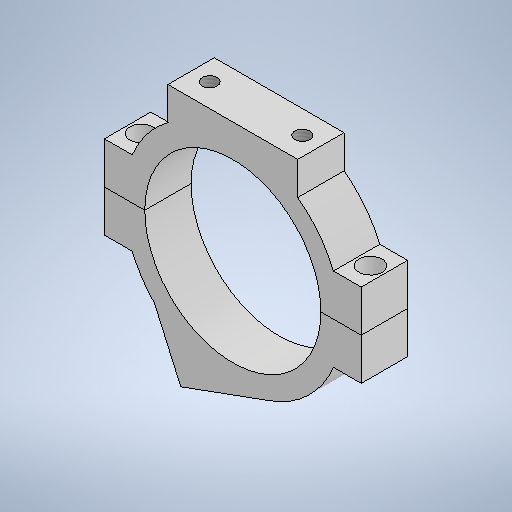
# Autodesk Inventor part: 2051
Saved by Autodesk Inventor 2025 (Build 290162010, 162A)
## iProperties
Created: 2024-06-01
Part Number: 2051
Material: Generic
Document SubType Name: Modeling
Designer: Fabri
Density: 1 g/cm^3
Appearance: Default
Author: Fabri
Autodesk Inventor part; units mm, degrees
ref_plane "YZ Plane" through (0, 0, 0) normal (1, 0, 0) x (0, 1, 0)
ref_plane "XZ Plane" through (0, 0, 0) normal (0, 1, 0) x (-1, 0, 0)
sketch "Sketch1" plane through (0, 0, 0) normal (0, 1, 0) x (-1, 0, 0)
  circle A0 centre (0, 0) radius 19
  arc A1 (16.9227, -16.3055) -> (-8.0375, -22.0828) centre (0, 0) ccw
  line L0 (0, 23.5) -> (0, -23.5) construction
  line L1 (23.5, 0) -> (-23.5, 0) construction
  line L2 (-8.0375, -22.0828) -> (11.2262, -29.0942)
  line L3 (11.2262, -29.0942) -> (16.9227, -16.3055)
  line L4 (0, 0) -> (-8.9052, -24.4669) construction
  line L5 (21.7083, 9) -> (27.7083, 9)
  line L6 (27.7083, 9) -> (27.7083, -9)
  line L7 (27.7083, -9) -> (21.7083, -9)
  line L8 (14, 18.8746) -> (14, 26)
  line L9 (14, 26) -> (-14, 26)
  line L10 (-14, 26) -> (-14, 18.8746)
  line L11 (-21.7083, 9) -> (-27.7083, 9)
  line L12 (-27.7083, 9) -> (-27.7083, -9)
  line L13 (-27.7083, -9) -> (-21.7083, -9)
  point P0 (-14, 22.4373)
  dimension "d1" = 47
  dimension "d0" = 20.5
  dimension "d2" = 38
  dimension "d5" = 20
  dimension "d7" = 14
  dimension "d8" = 18
  dimension "d9" = 6
  dimension "d10" = 28
  dimension "d11" = 18
  dimension "d32" = 6
  dimension "d33" = 17
  constraints: 28 end point, 6 perpendicular, 4 midpoint, 3 horizontal, 2 coincident, 2 vertical, 1 centre point, 1 point on line, 17 other
  measures "d0" distance of L2.start L2.end
  measures "d2" diameter of A0
  measures "d5" angle of L4 L0
  measures "d7" distance of L2.end L3.end
  measures "d8" distance between parallel lines of L7 L5
  measures "d9" distance of L5.start L5.end
  measures "d10" distance from line of point (-14, 22.437) L8
  measures "d11" distance of L11.end L12.end
  measures "d32" distance of L11.start L11.end
  measures "d33" distance from line of L5.start L9
extrude "Extrusion1" add sketch "Sketch1" along normal blind 10
sketch "Sketch2" plane through (-16.9227, 0, -16.3055) normal (-0.9135, 0, -0.4069) x (-0.4069, 0, 0.9135)
  line L0 (-14, 0) -> (-14, 10) projected
  point P0 (8.0089, 0)
  point P1 (-8, 3.373)
  dimension "d24" = 6
  measures "d24" distance from line of L0 point (-8, 3.373)
hole "Hole1" at (-13.6676, 3.373, -23.6133) direction (0.9135, 0, 0.4069) diameter 3 depth 9.5 counterbore diameter 5 counterbore depth 5
sketch "Sketch3" plane through (-21.7083, 0, -9) normal (0, 0, -1) x (-1, 0, 0)
  line L0 (6, 0) -> (6, 10) projected
  line L1 (0, 0) -> (6, 0) projected
  point P0 (-21.7083, 0)
  point P1 (3, 5)
  point P2 (6, 5)
  point P3 (3, 0)
  constraints: 2 midpoint, 1 horizontal alignment, 1 vertical alignment
hole "Hole2" at (-24.7083, 5, -9) direction (0, 0, 1) diameter 5 end through all
sketch "Sketch4" plane through (27.7083, 0, -9) normal (0, 0, -1) x (-1, 0, 0)
  line L0 (0, 0) -> (0, 10) projected
  line L1 (0, 0) -> (6, 0) projected
  point P0 (27.7083, 0)
  point P1 (3, 5)
  point P2 (0, 5)
  point P3 (3, 0)
  constraints: 2 midpoint, 1 horizontal alignment, 1 vertical alignment
hole "Hole3" at (24.7083, 5, -9) direction (0, 0, 1) diameter 5 end through all
sketch "Sketch5" plane through (-14, 0, 26) normal (0, 0, 1) x (1, 0, 0)
  line L0 (0, 0) -> (0, 10) projected
  line L1 (28, 0) -> (28, 10) projected
  point P0 (14, 0)
  point P1 (4, 5)
  point P2 (24, 5)
  point P3 (0, 5)
  point P4 (28, 5)
  dimension "d48" = 4
  dimension "d49" = 4
  constraints: 2 horizontal alignment, 2 midpoint
  measures "d48" distance from line of L0 point (4, 5)
  measures "d49" distance from line of L1 point (24, 5)
hole "Hole4" at (-10, 5, 26) at (10, 5, 26) direction (0, 0, -1) diameter 3.242 depth 6 thread size "M4x0.7" class "6H" standard "ISO Metric profile"
ref_plane "Work Plane1" through (0, 0, 0) normal (0, 0, 1) x (1, 0, 0)
split_face "Split1"
equation "\"d49\" = d48"
body "Solid1"
